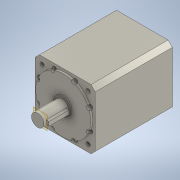
# Autodesk Inventor part: Caja reductora 1KW
Saved by Autodesk Inventor 2022.1 (Build 261234000, 234)
## iProperties
Created: 2021-09-10
Part Number: Caja reductora 1KW
Material: Generic
Document SubType Name: Sheet Metal
Designer: ARMU
Density: 1 g/cm^3
Sheet Metal Rule: Por defecto
Appearance: Acero - Fundido
Author: ARMU
Autodesk Inventor part; units mm, degrees
ref_plane "YZ Plane" through (0, 0, 0) normal (1, 0, 0) x (0, 1, 0)
ref_plane "XZ Plane" through (0, 0, 0) normal (0, 1, 0) x (-1, 0, 0)
ref_plane "XY Plane" through (0, 0, 0) normal (0, 0, 1) x (1, 0, 0)
sketch "Sketch1" plane through (0, 0, 0) normal (0, 0, 1) x (1, 0, 0)
  line L0 (-60, -60) -> (60, -60)
  line L1 (60, -60) -> (60, 60)
  line L2 (60, 60) -> (-60, 60)
  line L3 (-60, 60) -> (-60, -60)
  line L4 (-60, -60) -> (60, 60) construction
  line L5 (60, -60) -> (-60, 60) construction
  point P0 (0, 0)
  dimension "d0" = 120
  dimension "d1" = 120
  constraints: 12 end point, 2 midpoint, 2 parallel, 1 horizontal, 1 perpendicular
  measures "d0" distance of L2.end L1.end
  measures "d1" distance of L1.end L0.end
extrude "Extrusion1" add sketch "Sketch1" along normal blind 154
sketch "Sketch2" plane through (0, 0, 154) normal (0, 0, 1) x (1, 0, 0)
  circle A0 centre (0, 0) radius 55
  dimension "d4" = 110
  constraints: 1 centre point, 1 coincident
  measures "d4" diameter of A0
extrude "Extrusion2" add sketch "Sketch2" along normal blind 4
sketch "Sketch3" plane through (0, 0, 158) normal (0, 0, 1) x (1, 0, 0)
  circle A0 centre (0, 0) radius 17.5
  dimension "d7" = 35
  constraints: 1 centre point, 1 coincident
  measures "d7" diameter of A0
extrude "Extrusion3" add sketch "Sketch3" along normal blind 2
sketch "Sketch4" plane through (0, 0, 160) normal (0, 0, 1) x (1, 0, 0)
  circle A0 centre (0, 0) radius 12.5
  dimension "d10" = 25
  constraints: 1 centre point, 1 coincident
  measures "d10" diameter of A0
extrude "Extrusion4" add sketch "Sketch4" along normal blind 49
sketch "Sketch5" plane through (0, 0, 154) normal (0, 0, 1) x (1, 0, 0)
  line L0 (60, -60) -> (60, 60) construction
  line L1 (0, 0) -> (60, 60) construction
  circle A0 centre (45.9619, 45.9619) radius 4.25
  circle A1 centre (0, 0) radius 65 construction
  circle A2 centre (-45.9619, 45.9619) radius 4.25
  circle A3 centre (-45.9619, -45.9619) radius 4.25
  circle A4 centre (45.9619, -45.9619) radius 4.25
  dimension "d14" = 130
  dimension "d13" = 8.5
  dimension "d17" = 360
  constraints: 4 centre point, 2 end point, 1 coincident, 1 point on line, 12 other
  measures "d13" diameter of A0
extrude "Extrusion5" cut sketch "Sketch5" against normal blind 50
sketch "Sketch6" plane through (0, 0, 158) normal (0, 0, 1) x (1, 0, 0)
  circle A0 centre (50.8134, 21.0476) radius 4.25
  line L0 (0, 0) -> (64.336, 26.6488) construction
  line L1 (0, 0) -> (69.6368, 0) construction
  circle A1 centre (0, 0) radius 55 construction
  circle A2 centre (21.0476, 50.8134) radius 4.25
  circle A3 centre (-21.0476, 50.8134) radius 4.25
  circle A4 centre (-50.8134, 21.0476) radius 4.25
  circle A5 centre (-50.8134, -21.0476) radius 4.25
  circle A6 centre (-21.0476, -50.8134) radius 4.25
  circle A7 centre (21.0476, -50.8134) radius 4.25
  circle A8 centre (50.8134, -21.0476) radius 4.25
  dimension "d23" = 110
  dimension "d21" = 8.5
  dimension "d22" = 22.5
  dimension "d26" = 360
  constraints: 8 centre point, 4 end point, 1 coincident, 1 equal length, 1 horizontal, 1 point on line, 20 other
  measures "d21" diameter of A0
  measures "d22" angle of L1 L0
extrude "Extrusion6" cut sketch "Sketch6" against normal blind 50
ref_plane "Work Plane1" through (0, 0, 204) normal (0, 0, 1) x (1, 0, 0)
sketch "Sketch7" plane through (0, 0, 204) normal (0, 0, 1) x (1, 0, 0)
  line L0 (9.5, 4) -> (17.5, 4)
  line L1 (17.5, 4) -> (17.5, -4)
  line L2 (17.5, -4) -> (9.5, -4)
  line L3 (9.5, -4) -> (9.5, 4)
  line L4 (0, 0) -> (17.5, 0) construction
  circle A0 centre (0, 0) radius 17.5 construction
  line L5 (9.5, 4) -> (17.5, -4) construction
  line L6 (17.5, 4) -> (9.5, -4) construction
  point P0 (13.5, 0)
  point P1 (17.5, 0)
  dimension "d31" = 8
  dimension "d32" = 8
  constraints: 14 end point, 2 horizontal, 2 midpoint, 2 parallel, 2 point on circle, 1 perpendicular, 1 point on line
  measures "d31" distance of L1.end L2.end
  measures "d32" distance of L0.end L1.end
extrude "Extrusion7" add sketch "Sketch7" against normal blind 40
sketch "Sketch8" plane through (0, 0, 0) normal (0, 0, -1) x (-1, 0, 0)
  circle A0 centre (0, 0) radius 9.5
  dimension "d35" = 19
  constraints: 1 centre point, 1 coincident
  measures "d35" diameter of A0
extrude "Extrusion8" cut sketch "Sketch8" against normal blind 40
sketch "Sketch9" plane through (0, 0, 0) normal (0, 0, -1) x (-1, 0, 0)
  circle A0 centre (0, 0) radius 47.5
  dimension "d38" = 95
  constraints: 1 centre point, 1 coincident
  measures "d38" diameter of A0
extrude "Extrusion9" cut sketch "Sketch9" against normal blind 3
sketch "Sketch10" plane through (0, 0, 0) normal (0, 0, -1) x (-1, 0, 0)
  circle A0 centre (0, 0) radius 62.5 construction
  line L0 (60, 60) -> (60, -60) construction
  line L1 (0, 0) -> (60, 60) construction
  circle A1 centre (44.1942, 44.1942) radius 4.75
  circle A2 centre (-44.1942, 44.1942) radius 4.75
  circle A3 centre (-44.1942, -44.1942) radius 4.75
  circle A4 centre (44.1942, -44.1942) radius 4.75
  dimension "d41" = 125
  dimension "d42" = 9.5
  dimension "d45" = 360
  constraints: 4 centre point, 2 end point, 1 coincident, 1 point on line, 12 other
  measures "d42" diameter of A1
extrude "Extrusion10" cut sketch "Sketch10" against normal blind 50
chamfer "Chamfer1" distance 8.5 angle 45 4 edges at (60, 60, 77) (-60, 60, 77) (-60, -60, 77) (60, -60, 77)
equation "\"BendRadius\" = Thickness"
equation "\"BendReliefWidth\" = Thickness"
equation "\"BendReliefDepth\" = 0.5 * Thickness"
equation "\"CornerReliefSize\" = 4 * Thickness"
equation "\"MinimumRemnant\" = 2 * Thickness"
equation "\"TransitionRadius\" = BendRadius"
equation "\"JacobiRadiusSize\" = BendRadius"
equation "\"GapSize\" = Thickness"
equation "\"Thickness\" = 3.048"
body "Solid1"
